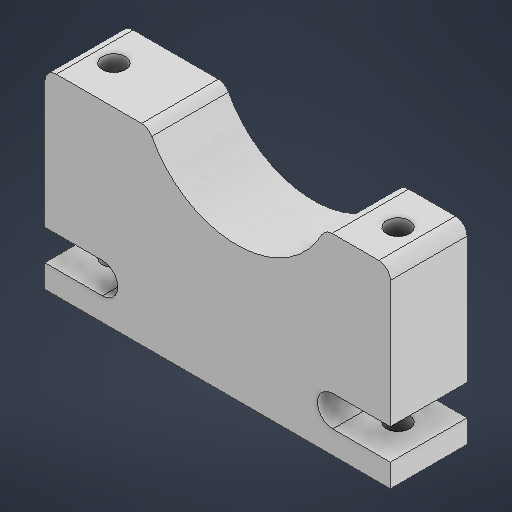
# Autodesk Inventor part: součást 1
Saved by Autodesk Inventor 2025.1 (Build 291241000, 241)
## iProperties
Created: 2025-04-28
Part Number: součást 1
Material: Všeobecné
Document SubType Name: Modeling
Designer: Dominik Petříček
Density: 1 g/cm^3
Appearance: Výchozí
Author: Dominik Petříček
Autodesk Inventor part; units mm, degrees
ref_plane "YZ Plane" through (0, 0, 0) normal (1, 0, 0) x (0, 1, 0)
ref_plane "XZ Plane" through (0, 0, 0) normal (0, 1, 0) x (-1, 0, 0)
ref_plane "XY Plane" through (0, 0, 0) normal (0, 0, 1) x (1, 0, 0)
sketch "Náčrt1" plane through (0, 0, 0) normal (0, 0, 1) x (1, 0, 0)
  line L0 (0, 0) -> (90, 0)
  line L1 (90, 0) -> (90, 6)
  line L2 (90, 6) -> (75, 6)
  arc A0 (75, 14) -> (75, 6) centre (75, 10) ccw
  line L3 (75, 14) -> (90, 14)
  line L4 (0, 0) -> (0, 6)
  line L5 (0, 6) -> (15, 6)
  arc A1 (15, 6) -> (15, 14) centre (15, 10) ccw
  line L6 (15, 14) -> (0, 14)
  line L7 (15, 14) -> (30, 14) construction
  line L8 (90, 47) -> (90, 14)
  line L9 (0, 47) -> (0, 14)
  arc A2 (3, 50) -> (0, 47) centre (3, 47) ccw
  arc A3 (90, 47) -> (87, 50) centre (87, 47) ccw
  arc A4 (27.8579, 48.3929) -> (72.1421, 48.3929) centre (50, 60) ccw
  line L10 (3, 50) -> (25.2008, 50)
  line L11 (74.7992, 50) -> (87, 50)
  arc A5 (27.8579, 48.3929) -> (25.2008, 50) centre (25.2008, 47) ccw
  arc A6 (74.7992, 50) -> (72.1421, 48.3929) centre (74.7992, 47) ccw
  point P0 (72.9129, 50)
  point P1 (27.0871, 50)
  dimension "d0" = 90
  dimension "d1" = 6
  dimension "d4" = 15
  dimension "d5" = 6
  dimension "d9" = 15
  dimension "d10" = 180
  dimension "d13" = 3
  dimension "d16" = 50
  dimension "d17" = 3
  constraints: 24 end point, 16 point on circle, 11 tangent, 7 centre point, 4 horizontal, 4 perpendicular, 2 equal radius, 2 point on line, 2 vertical, 1 collinear
  measures "d0" distance of L0.start L0.end
  measures "d1" distance of L0.end L1.end
  measures "d4" distance of L3.start L3.end
  measures "d5" distance of L0.start L4.end
  measures "d9" distance of L6.start L6.end
  measures "d10" angle of L6 L7
  measures "d13" radius of A2
  measures "d16" diameter of A4
  measures "d17" radius of A5
extrude "Vysunutí1" add sketch "Náčrt1" along normal blind 20
sketch "Náčrt2" plane through (3, 50, 0) normal (0, 1, 0) x (1, 0, 0)
  line L0 (-3, -20) -> (87, -20) projected
  line L1 (-3, -20) -> (5, -20)
  line L2 (5, -20) -> (5, -10)
  line L3 (5, -20) -> (15, -20) construction
  line L4 (87, -20) -> (79, -20)
  line L5 (79, -20) -> (79, -10)
  circle A0 centre (79, -10) radius 3
  circle A1 centre (5, -10) radius 3
  point P0 (-3, 0)
  dimension "d20" = 8
  dimension "d21" = 10
  dimension "d22" = 90
  dimension "d23" = 8
  dimension "d24" = 10
  dimension "d25" = 90
  dimension "d26" = 6
  dimension "d27" = 6
  constraints: 10 end point, 2 centre point, 2 coincident, 2 perpendicular, 2 point on line, 1 horizontal, 1 vertical
  measures "d20" distance of L0.start L1.end
  measures "d21" distance of L1.end L2.end
  measures "d22" angle of L3 L2
  measures "d23" distance of L0.end L4.end
  measures "d24" distance of L4.end L5.end
  measures "d25" angle of L4 L5
  measures "d26" diameter of A0
  measures "d27" diameter of A1
extrude "Vysunutí2" cut sketch "Náčrt2" against normal through all
